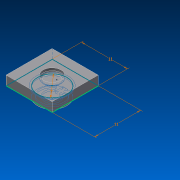
# Autodesk Inventor part: power button
Saved by Autodesk Inventor 2015 (Build 190159000, 159)
## iProperties
Created: 2017-03-16
Part Number: power button
Material: Generic
Document SubType Name: Modeling
Designer: ZigZagJoe
Density: 1 g/cm^3
Appearance: Default
Author: ZigZagJoe
Autodesk Inventor part; units mm, degrees
ref_plane "YZ Plane" through (0, 0, 0) normal (1, 0, 0) x (0, 1, 0)
ref_plane "XZ Plane" through (0, 0, 0) normal (0, 1, 0) x (-1, 0, 0)
ref_plane "XY Plane" through (0, 0, 0) normal (0, 0, 1) x (1, 0, 0)
sketch "Sketch1" plane through (0, 0, 0) normal (0, 0, 1) x (1, 0, 0)
  line L0 (-4.7979, 3.7252) -> (6.2021, 3.7252)
  line L1 (6.2021, 3.7252) -> (6.2021, -7.2748)
  line L2 (6.2021, -7.2748) -> (-4.7979, -7.2748)
  line L3 (-4.7979, -7.2748) -> (-4.7979, 3.7252)
  circle A0 centre (0.7021, -1.7748) radius 3.5
  point P0 (0, 0)
  dimension "d0" = 11
  dimension "d1" = 11
  dimension "d2" = 7
  constraints: 8 end point, 2 parallel, 1 centre point, 1 horizontal, 1 perpendicular
  measures "d0" distance of L0.start L0.end
  measures "d1" distance of L0.end L1.end
  measures "d2" diameter of A0
extrude "Extrusion1" add sketch "Sketch1" along normal blind 2.2 contours L0 L1 L2 L3 | A0
extrude "Extrusion2" add sketch "Sketch1" against normal blind 2.4 contours A0
sketch "Sketch2" plane through (0, 0, 2.2) normal (0, 0, 1) x (1, 0, 0)
  circle A0 centre (0.7021, -1.7748) radius 2.125
  line L0 (6.2021, 3.7252) -> (-4.7979, 3.7252) projected
  line L1 (-4.7979, 3.7252) -> (-4.7979, -7.2748) projected
  point P0 (0, 0)
  dimension "d7" = 4.25
  dimension "d8" = 5.5
  dimension "d9" = 5.5
  constraints: 1 centre point
  measures "d7" diameter of A0
  measures "d8" distance from line of A0.centre L0
  measures "d9" distance from line of L1 A0.centre
extrude "Extrusion3" cut sketch "Sketch2" against normal blind 1
fillet "Fillet1" radius 0.4 1 edges at (-1.4229, -1.7748, 1.2)
fillet "Fillet2" radius 0.4 1 edges at (-2.7979, -1.7748, 0)
sketch "Sketch3" plane through (0.7021, -1.7748, -2.4) normal (0, 0, -1) x (-1, 0, 0)
  arc A0 (-1.4, 2.4249) -> (1.4, 2.4249) centre (0, 0) ccw
  line L0 (0, 0) -> (-1.4, 2.4249) construction
  line L1 (0, 0) -> (1.4, 2.4249) construction
  arc A1 (-0.9, 1.5588) -> (0.9, 1.5588) centre (0, 0) ccw
  line L2 (0, 0) -> (-0.9, 1.5588) construction
  line L3 (0, 0) -> (0.9, 1.5588) construction
  line L4 (-5.5, 5.5) -> (-5.5, -5.5) projected
  line L5 (5.5, 5.5) -> (-5.5, 5.5) projected
  line L6 (-1.4, 2.4249) -> (-0.9, 1.5588)
  line L7 (0.9, 1.5588) -> (1.4, 2.4249)
  line L8 (5.5, -5.5) -> (5.5, 5.5) projected
  line L9 (-0.5, 3.1) -> (0.5, 3.1)
  line L10 (0.5, 3.1) -> (0.5, 1.3)
  line L11 (0.5, 1.3) -> (-0.5, 1.3)
  line L12 (-0.5, 1.3) -> (-0.5, 3.1)
  point P0 (0.7021, 1.7748)
  dimension "d17" = 2.8
  dimension "d18" = 60
  dimension "d19" = 1.8
  dimension "d20" = 60
  dimension "d21" = 5.5
  dimension "d22" = 5.5
  dimension "d23" = 30
  dimension "d24" = 1
  dimension "d25" = 0.5
  dimension "d26" = 1.8
  dimension "d27" = 1.3
  constraints: 20 end point, 4 point on circle, 2 centre point, 2 parallel, 1 coincident, 1 collinear, 1 horizontal, 1 perpendicular, 1 point on line
  measures "d17" radius of A0
  measures "d18" angle of L1 L0
  measures "d19" radius of A1
  measures "d20" angle of L3 L2
  measures "d21" distance from line of L4 L0.start
  measures "d22" distance from line of L5 L0.start
  measures "d23" angle of L8 L0
  measures "d24" distance of L10.end L11.end
  measures "d25" distance from line of L12 L0.start
  measures "d26" distance between parallel lines of L11 L9
  measures "d27" distance from line of L0.start L11
extrude "Extrusion4" cut sketch "Sketch3" against normal blind 0.4
equation "\"d18\" = d20"
equation "\"d23\" = 0.5 * d20"
equation "\"d25\" = 0.5 * d24"
body "Solid1"
